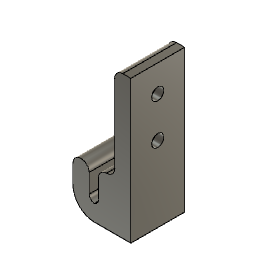
model (Autodesk Fusion 360 design; units mm, degrees)
Autodesk Fusion 360 part; units mm, degrees
note: some values were not read from the file. Set by a fixed rule: which sketch regions a step uses.
sketch "Sketch1" plane through (0, 0, 0) normal (0, 1, 0) x (1, 0, 0)
  line L0 (6, -18) -> (6, -6)
  line L1 (6, -6) -> (9.5, -6)
  line L2 (9.5, -6) -> (9.5, -18)
  line L3 (15.5, -53) -> (21.5, -53)
  line L4 (21.5, -53) -> (21.5, 0)
  line L5 (21.5, 0) -> (0, 0)
  line L6 (0, 0) -> (0, -18)
  line L7 (0, -18) -> (6, -18)
  line L8 (9.5, -18) -> (15.5, -18)
  line L9 (15.5, -18) -> (15.5, -53)
  dimension "d1" = 12
  dimension "d2" = 3.5
  dimension "d4" = 6
  dimension "d5" = 6
  dimension "d6" = 35
  dimension "d31" = 6
  dimension "d32" = 12
  constraint vertical L0
  constraint perpendicular L0 L1
  constraint perpendicular L1 L2
  constraint perpendicular L2 L3
  constraint perpendicular L3 L4
  constraint coincident L5.end L6.start
  constraint perpendicular L2 L5
  constraint perpendicular L5 L6
  constraint perpendicular L6 L7
  constraint perpendicular L2 L8
  constraint perpendicular L3 L9
  constraint collinear L7 L8
  measures "d1" distance of L0.start L0.end
  measures "d2" distance of L0.end L1.end
  measures "d4" distance of L0.start L6.end
  measures "d5" distance of L1 L5
  measures "d6" distance of L3 L7
  measures "d31" distance of L4 L9
  measures "d32" distance of L2 L4
extrude "Extrude1" add sketch "Sketch1" along normal blind 20
sketch "Sketch2" plane through (15.5, 0, 0) normal (-1, 0, 0) x (0, -1, 0)
  line L0 (0, 6) -> (0, 53)
  line L1 (-20, 18) -> (-20, 6)
  line L2 (-20, 6) -> (0, 6)
  circle A0 centre (-10, 43) radius 5
  circle A1 centre (-10, 28) radius 5
  line L3 (-20, 53) -> (-10, 43) construction
  line L4 (-10, 43) -> (0, 53) construction
  line L5 (-10, 43) -> (-10, 28) construction
  circle A2 centre (-10, 43) radius 2.25
  circle A3 centre (-10, 28) radius 2.25
  line L6 (0, 18) -> (-20, 18)
  line L7 (0, 18) -> (0, 53)
  line L8 (0, 53) -> (-20, 53)
  line L9 (-20, 53) -> (-20, 18)
  line L10 (-20, 18) -> (0, 18)
  dimension "d9" = 10
  dimension "d11" = 15
  dimension "d12" = 10
  dimension "d13" = 10
  dimension "d14" = 4.5
  dimension "d15" = 4.5
  constraint coincident A0.centre L3.end
  constraint coincident A1.centre L5.end
  constraint vertical L5
  constraint equal L3 L4
  constraint concentric A0 A2
  constraint concentric A1 A3
  constraint coincident L3.start L8.end
  constraint coincident L0.end L4.end
  measures "d9" diameter of A0
  measures "d11" distance of A0.centre A1.centre
  measures "d12" vertical distance of A0.centre L3.start
  measures "d13" diameter of A1
  measures "d14" diameter of A2
  measures "d15" diameter of A3
extrude "Extrude2" cut sketch "Sketch2" against normal up to surface (6 mm away) contours A2 | A3
fillet "Fillet2" radius 8 1 edges at (0, 10, 0)
fillet "Fillet2" radius 3 3 edges at (15.5, 10, 53) (15.5, 10, 18) (9.5, 10, 18)
fillet "Fillet2" radius 3 2 edges at (0, 10, 18) (6, 10, 18)
fillet "Fillet2" radius 2 2 edges at (6, 10, 6) (9.5, 10, 6)
chamfer "Chamfer2" distance 3 angle 45 2 edges at (15.5, 12.0977, 43.8136) (15.5, 12.0977, 28.8136)
ref_plane "WorkPlane1" through (3, 10.8689, 18) normal (0, 0, 1) x (-1, 0, 0)
equation "d13 = d9"
equation "d15 = d14"
